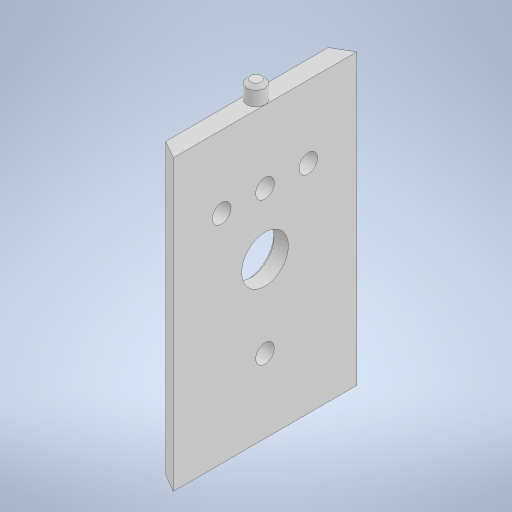
# Autodesk Inventor part: col_face_mic
Saved by Autodesk Inventor 2024 (Build 280153000, 153)
## iProperties
Created: 2024-03-18
Part Number: col_face_mic
Material: 일반
Document SubType Name: Modeling
Designer: SSAFY
Density: 1 g/cm^3
Appearance: 기본값
Author: SSAFY
Autodesk Inventor part; units mm, degrees
ref_plane "YZ Plane" through (0, 0, 0) normal (1, 0, 0) x (0, 1, 0)
ref_plane "XZ Plane" through (0, 0, 0) normal (0, 1, 0) x (-1, 0, 0)
ref_plane "XY Plane" through (0, 0, 0) normal (0, 0, 1) x (1, 0, 0)
sketch "스케치2" plane through (0, 0, 0) normal (0, 1, 0) x (-1, 0, 0)
  line L0 (0, 45) -> (38.9711, 22.5)
  line L1 (38.9711, 22.5) -> (38.9711, -22.5)
  line L2 (38.9711, -22.5) -> (0, -45)
  line L3 (0, -45) -> (-38.9711, -22.5)
  line L4 (-38.9711, -22.5) -> (-38.9711, 22.5)
  line L5 (-38.9711, 22.5) -> (0, 45)
  line L6 (0, 50.7735) -> (43.9711, 25.3868)
  line L7 (43.9711, 25.3868) -> (43.9711, -25.3868)
  line L8 (43.9711, -25.3868) -> (0, -50.7735)
  line L9 (0, -50.7735) -> (-43.9711, -25.3868)
  line L10 (-43.9711, -25.3868) -> (-43.9711, 25.3868)
  line L11 (-43.9711, 25.3868) -> (0, 50.7735)
  line L12 (-43.9711, 25.3868) -> (-38.9711, 22.5)
  line L13 (-38.9711, -22.5) -> (-43.9711, -25.3868)
  point P0 (0, 0)
  point P1 (0, 0)
  dimension "d0" = 45
  dimension "d1" = 5
  constraints: 28 end point, 1 coincident, 18 other
  measures "d0" distance of L3.end L4.end
  measures "d1" distance between parallel lines of L4 L10
extrude "돌출1" add sketch "스케치2" along normal blind 80 contours L4 L13 L10 L12
sketch "스케치3" plane through (38.9711, 0, -22.5) normal (-1, 0, 0) x (0, 0, 1)
  line L0 (0, 0) -> (45, 0) construction
  circle A0 centre (22.5, 20.4) radius 2.6
  point P0 (22.5, 0)
  point P1 (22.5, 0)
  dimension "d4" = 5.2
  dimension "d5" = 20.4
  constraints: 1 centre point, 1 midpoint
  measures "d4" diameter of A0
  measures "d5" distance of point (22.5, 0) A0.centre
extrude "돌출2" cut sketch "스케치3" against normal through all
sketch "스케치4" plane through (0, 80, 0) normal (0, 1, 0) x (1, 0, 0)
  line L0 (38.9711, 22.5) -> (38.9711, -22.5) construction
  circle A0 centre (41.4711, 0) radius 2.5
  point P0 (0, 0)
  dimension "d8" = 5
  constraints: 1 centre point, 1 tangent
  measures "d8" diameter of A0
extrude "돌출3" add sketch "스케치4" along normal blind 5
sketch "스케치5" plane through (43.9711, 0, 25.3868) normal (1, 0, 0) x (0, 0, -1)
  line L0 (50.7735, 0) -> (50.7735, 80) construction
  line L1 (25.3868, 80) -> (50.7735, 80) construction
  line L2 (0, 0) -> (0, 80) construction
  circle A0 centre (25.3868, 60) radius 2.6
  circle A1 centre (13.3868, 60) radius 2.6
  circle A2 centre (37.3868, 60) radius 2.6
  line L3 (0, 60) -> (50.7735, 60)
  point P0 (25.3868, 0)
  dimension "d11" = 20
  dimension "d12" = 0
  dimension "d13" = 0
  dimension "d14" = 0
  dimension "d15" = 12
  dimension "d16" = 12
  dimension "d17" = 5.2
  dimension "d18" = 5.2
  dimension "d19" = 5.2
  constraints: 3 centre point, 2 end point, 2 point on line, 1 horizontal, 1 midpoint
  measures "d11" distance between parallel lines of L1 L3
  measures "d12" distance from line of A1.centre L3
  measures "d13" distance from line of A0.centre L3
  measures "d14" distance from line of A2.centre L3
  measures "d15" distance of point (25.387, 60) A1.centre
  measures "d16" distance of A2.centre A0.centre
  measures "d17" diameter of A0
  measures "d18" diameter of A1
  measures "d19" diameter of A2
extrude "돌출4" cut sketch "스케치5" against normal through all
sketch "스케치6" plane through (43.9711, 0, 25.3868) normal (1, 0, 0) x (0, 0, -1)
  line L0 (0, 0) -> (50.7735, 0) construction
  circle A0 centre (25.3868, 43) radius 6.5
  point P0 (25.3868, 0)
  dimension "d22" = 13
  dimension "d23" = 43
  constraints: 1 centre point
  measures "d22" diameter of A0
  measures "d23" distance from line of L0 A0.centre
extrude "돌출5" cut sketch "스케치6" against normal through all
chamfer "모따기1" distance 1 angle 45 6 edges at (38.9711, 85, 0) (38.9711, 60, -9.4) (38.9711, 60, 2.6) (38.9711, 60, 14.6) (38.9711, 43, 6.5) (38.9711, 20.4, -2.6)
